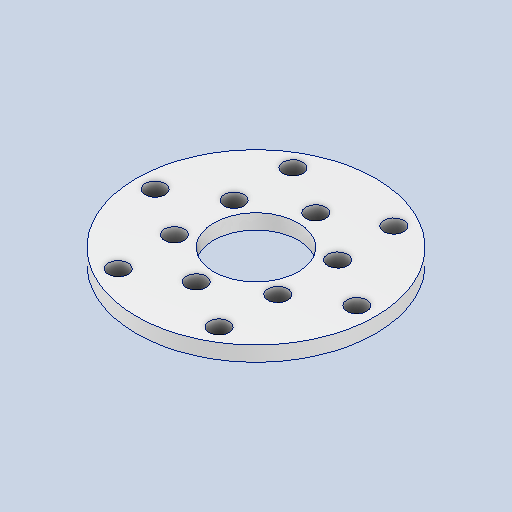
# Autodesk Inventor part: sholder_joint_s
Saved by Autodesk Inventor 2024.1 (Build 281209000, 209)
## iProperties
Created: 2024-02-14
Part Number: sholder_joint_s
Material: アルミニウム 6061
Document SubType Name: Sheet Metal
Designer: hibik
Density: 2.7 g/cm^3
Sheet Metal Rule: Default_mm
Appearance: アルミニウム - フラット
Author: hibik
Autodesk Inventor part; units mm, degrees
ref_plane "YZ Plane" through (0, 0, 0) normal (1, 0, 0) x (0, 1, 0)
ref_plane "XZ Plane" through (0, 0, 0) normal (0, 1, 0) x (-1, 0, 0)
ref_plane "XY Plane" through (0, 0, 0) normal (0, 0, 1) x (1, 0, 0)
sketch "スケッチ1" plane through (0, 0, 0) normal (0, 1, 0) x (-1, 0, 0)
  circle A0 centre (0, 0) radius 8.25 construction
  circle A1 centre (0, 0) radius 12
  circle A2 centre (0, 0) radius 10.125 construction
  circle A3 centre (10.125, 0) radius 1
  line L0 (16.8, 0) -> (-16.8, 0)
  circle A4 centre (5.0625, 8.7685) radius 1
  circle A5 centre (-5.0625, 8.7685) radius 1
  circle A6 centre (-10.125, 0) radius 1
  circle A7 centre (-5.0625, -8.7685) radius 1
  circle A8 centre (5.0625, -8.7685) radius 1
  circle A9 centre (0, 0) radius 4.25
  dimension "d3" = 20.25
  dimension "d0" = 16.5
  dimension "d1" = 24
  dimension "d4" = 2
  dimension "d7" = 360
  dimension "d9" = 8.5
  measures "d0" diameter of A0
  measures "d1" diameter of A1
  measures "d4" diameter of A3
  measures "d9" diameter of A9
extrude "プレート1" add sketch "スケッチ1" along normal blind 1.5 contours L0 A3 A9 A6 A1 | A1 L0 A6 A9 A3
sketch "スケッチ2" plane through (0, 0, 0) normal (0, -1, 0) x (1, 0, 0)
  circle A0 centre (5.1962, -3) radius 1 projected
  circle A1 centre (5.1962, 3) radius 1 projected
  circle A2 centre (0, 6) radius 1 projected
  circle A3 centre (-5.1962, 3) radius 1 projected
  line L0 (16, 8) -> (16, -8) projected
  line L1 (-16, -8) -> (-9.798, -8) projected
  arc A4 (-8.3983, -8.5714) -> (8.3983, -8.5714) centre (0, 0) ccw projected
  line L2 (9.798, -8) -> (16, -8) projected
  line L3 (-16, -8) -> (-16, 8) projected
  line L4 (16, 8) -> (9.798, 8) projected
  arc A5 (8.3983, 8.5714) -> (-8.3983, 8.5714) centre (0, 0) ccw projected
  line L5 (-9.798, 8) -> (-16, 8) projected
  circle A6 centre (-5.1962, 3) radius 1 projected
  circle A7 centre (-5.1962, -3) radius 1 projected
  circle A8 centre (0, 0) radius 4.25 projected
  circle A9 centre (0, -6) radius 1 projected
  circle A10 centre (5.1962, -3) radius 1 projected
  circle A11 centre (5.1962, 3) radius 1 projected
  circle A12 centre (0, 6) radius 1 projected
  circle A13 centre (0, -6) radius 1 projected
  circle A14 centre (-5.0625, 8.7685) radius 1 projected
  circle A15 centre (-5.0625, -8.7685) radius 1 projected
  circle A16 centre (10.125, 0) radius 1 projected
  circle A17 centre (5.0625, -8.7685) radius 1 projected
  circle A18 centre (-10.125, 0) radius 1 projected
  circle A19 centre (5.0625, 8.7685) radius 1 projected
  arc A20 (9.798, -8) -> (8.3983, -8.5714) centre (9.798, -10) ccw projected
  arc A21 (-8.3983, -8.5714) -> (-9.798, -8) centre (-9.798, -10) ccw projected
  arc A22 (-9.798, 8) -> (-8.3983, 8.5714) centre (-9.798, 10) ccw projected
  arc A23 (8.3983, 8.5714) -> (9.798, 8) centre (9.798, 10) ccw projected
  point P0 (0, 0)
  point P1 (0, 0)
  point P2 (0, 0)
extrude "切り取り1" cut sketch "スケッチ2" against normal blind 1.5 contours A0 | A1 | A2 | A3 | A7 | A9
equation "\"d3\" = 0.5 * d0 + 0.5 * d1"
equation "\"d10\" = Thickness"
equation "\"d2\" = Thickness"
equation "\"BendRadius\" = Thickness"
equation "\"BendReliefWidth\" = Thickness"
equation "\"BendReliefDepth\" = 0.5 * Thickness"
equation "\"CornerReliefSize\" = 4 * Thickness"
equation "\"MinimumRemnant\" = 2 * Thickness"
equation "\"TransitionRadius\" = BendRadius"
equation "\"JacobiRadiusSize\" = BendRadius"
equation "\"GapSize\" = Thickness"
equation "\"Thickness\" = 1.5"
